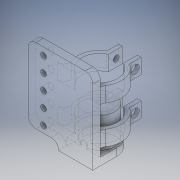
# Autodesk Inventor part: left_motor_mount
Saved by Autodesk Inventor 2018 (Build 220112000, 112)
## iProperties
Created: 2018-03-01
Part Number: left_motor_mount
Material: Generic
Document SubType Name: Modeling
Designer: njcfu
Density: 1 g/cm^3
Appearance: Default
Author: njcfu
Autodesk Inventor part; units mm, degrees
ref_plane "YZ Plane" through (0, 0, 0) normal (1, 0, 0) x (0, 1, 0)
ref_plane "XZ Plane" through (0, 0, 0) normal (0, 1, 0) x (-1, 0, 0)
sketch "Sketch1" plane through (0, 0, 0) normal (0, 1, 0) x (-1, 0, 0)
  circle A0 centre (0, 0) radius 12.7
  dimension "d0" = 25.4
  constraints: 1 centre point, 1 coincident
  measures "d0" diameter of A0
extrude "Extrusion1" add sketch "Sketch1" along normal blind 25.4
ref_plane "Work Plane1" through (0, 0, 12.7) normal (0, 0, 1) x (1, 0, 0)
sketch "Sketch3" plane through (0, 0, 12.7) normal (0, 0, 1) x (1, 0, 0)
  line L0 (-2.5, 0) -> (2.5, 0)
  line L1 (2.5, 0) -> (2.5, 2.4)
  line L2 (2.5, 2.4) -> (-2.5, 2.4)
  line L3 (-2.5, 2.4) -> (-2.5, 0)
  arc A0 (2.5, 2.4) -> (-2.5, 2.4) centre (0, 2.4) ccw
  point P0 (0, 0)
  dimension "d8" = 2.4
  dimension "d9" = 5
  dimension "d10" = 2.5
  dimension "d11" = 2.4
  constraints: 8 end point, 2 parallel, 2 point on circle, 1 centre point, 1 horizontal, 1 midpoint, 1 perpendicular
  measures "d8" distance of L2.end L0.start
  measures "d9" distance of L0.start L0.end
  measures "d10" distance from line of point (0, 0) L3
  measures "d11" distance from line of L2 point (0, 0)
extrude "Extrusion2" add sketch "Sketch3" along normal mid plane 2
sketch "Sketch4" plane through (0, 0, 0) normal (0, -1, 0) x (1, 0, 0)
  line L0 (14.2875, 20.05) -> (-14.2875, 20.05)
  line L1 (-14.2875, 20.05) -> (-14.2875, 0)
  line L2 (14.2875, 0) -> (14.2875, 20.05)
  arc A0 (-14.2875, 0) -> (14.2875, 0) centre (0, 0) ccw
  line L3 (-2.5, 13.7) -> (2.5, 13.7) projected
  arc A1 (-14.2875, 0) -> (14.2875, 0) centre (0, 0) ccw
  line L4 (0, 26.9175) -> (0, -21.155) projected
  circle A2 centre (0, 0) radius 12.7 projected
  dimension "d14" = 6.35
  dimension "d17" = 28.575
  dimension "d18" = 14.2875
  dimension "d19" = 14.2875
  dimension "d20" = 1.5875
  dimension "d21" = 28.575
  constraints: 6 end point, 4 point on circle, 2 centre point, 1 coincident, 1 concentric, 1 horizontal, 1 parallel, 1 perpendicular
  measures "d14" distance between parallel lines of L0 L3
  measures "d17" distance of L0.start L0.end
  measures "d18" distance between parallel lines of L4 L1
  measures "d19" radius of A0
  measures "d20" radial gap between concentric circles of A2 A0
  measures "d21" distance of L2.start L1.end
extrude "Extrusion3" add sketch "Sketch4" along normal blind 6.35
sketch "Sketch5" plane through (0, 0, 0) normal (0, 1, 0) x (1, 0, 0)
  line L0 (-39.6875, -20.05) -> (-39.6875, -13.7)
  line L1 (14.2875, 0) -> (14.2875, -20.05) projected
  line L2 (-39.6875, -20.05) -> (14.2875, -20.05)
  line L3 (14.2875, -20.05) -> (14.2875, -13.7)
  line L4 (14.2875, -13.7) -> (-39.6875, -13.7)
  line L5 (-39.6875, -13.7) -> (-39.6875, -20.05)
  point P0 (0, 0)
  dimension "d22" = 6.35
  dimension "d73" = 53.975
  dimension "d74" = 13.7
  constraints: 10 end point, 2 parallel, 1 horizontal, 1 point on line
  measures "d22" distance between parallel lines of L2 L4
  measures "d73" distance between parallel lines of L0 L1
  measures "d74" distance from line of L1.start L4
extrude "Extrusion4" add sketch "Sketch5" along normal blind 62.7634
ref_plane "Work Plane2" through (0, 12.7, 0) normal (0, -1, 0) x (1, 0, 0)
sketch "Sketch6" plane through (0, 12.7, 0) normal (0, -1, 0) x (1, 0, 0)
  arc A0 (6.35, -13.7142) -> (-6.35, -13.7142) centre (0, 0) ccw
  line L0 (-9.525, -25.4) -> (-9.525, -15.6117)
  line L1 (-4.445, -6.1638) -> (-1.27, -6.1638)
  line L2 (-6.35, -13.7142) -> (-6.35, -25.4)
  line L3 (-6.35, -25.4) -> (-9.525, -25.4)
  line L4 (6.35, -25.4) -> (6.35, -13.7142)
  line L5 (1.6345, -8.3094) -> (4.8095, -8.3094)
  line L6 (9.525, -25.4) -> (6.35, -25.4)
  line L7 (9.525, -15.6117) -> (9.525, -25.4)
  arc A1 (9.525, -15.6117) -> (-9.525, -15.6117) centre (0, 0) ccw
  arc A2 (-14.2875, 0) -> (14.2875, 0) centre (0, 0) ccw projected
  dimension "d26" = 30.226
  dimension "d27" = 3.175
  dimension "d28" = 9.525
  dimension "d29" = 25.4
  dimension "d30" = 3.175
  dimension "d31" = 17.0906
  dimension "d32" = 19.2362
  dimension "d33" = 4.7625
  dimension "d34" = 4.7155
  dimension "d35" = 7.8905
  dimension "d36" = 10.795
  dimension "d37" = 13.97
  constraints: 16 end point, 4 parallel, 4 point on circle, 2 centre point, 2 coincident, 2 equal length, 2 perpendicular, 1 collinear, 1 concentric
  measures "d26" diameter of A0
  measures "d27" distance of L2.end L0.start
  measures "d28" distance from line of point (0, 0) L0
  measures "d29" distance from line of point (0, 0) L3
  measures "d30" radial gap between concentric circles of A0 A1
  measures "d31" distance between parallel lines of L6 L5
  measures "d32" distance between parallel lines of L6 L1
  measures "d33" distance from line of A2.end L7
  measures "d34" distance from line of L5.end L7
  measures "d35" distance from line of L5.start L7
  measures "d36" distance from line of L1.end L7
  measures "d37" distance from line of L1.start L7
extrude "Extrusion5" add sketch "Sketch6" along normal mid plane 12.7
pattern_linear "Rectangular Pattern1" count 2 spacing 31.75 along (0, 1, 0) of "Extrusion5"
sketch "Sketch7" plane through (9.525, 38.1, -15.6117) normal (1, 0, 0) x (0, 0, -1)
  circle A0 centre (4.7083, 6.35) radius 2.4638
  circle A1 centre (4.7083, -25.4) radius 2.4638
  line L0 (9.7883, -31.75) -> (0, -31.75) projected
  line L1 (9.7883, 0) -> (0, 0) projected
  line L2 (9.7883, 12.7) -> (9.7883, 0) projected
  line L3 (9.7883, -19.05) -> (9.7883, -31.75) projected
  point P0 (-15.6117, -38.1)
  dimension "d43" = 4.9276
  dimension "d44" = 4.9276
  dimension "d45" = 6.35
  dimension "d46" = 6.35
  dimension "d47" = 5.08
  dimension "d48" = 5.08
  constraints: 2 centre point
  measures "d43" diameter of A0
  measures "d44" diameter of A1
  measures "d45" distance from line of L0 A1.centre
  measures "d46" distance from line of L1 A0.centre
  measures "d47" distance from line of L2 A0.centre
  measures "d48" distance from line of L3 A1.centre
extrude "Extrusion6" cut sketch "Sketch7" against normal through all
sketch "Sketch8" plane through (9.525, 38.1, -15.6117) normal (1, 0, 0) x (0, 0, -1)
  circle A0 centre (4.7083, 6.35) radius 3.4798
  circle A1 centre (4.7083, -25.4) radius 3.4798
  circle A2 centre (4.7083, 6.35) radius 2.4638 projected
  circle A3 centre (4.7083, -25.4) radius 2.4638 projected
  point P0 (-15.6117, -38.1)
  dimension "d51" = 6.9596
  dimension "d52" = 6.9596
  constraints: 2 centre point, 2 concentric
  measures "d51" diameter of A0
  measures "d52" diameter of A1
extrude "Extrusion7" cut sketch "Sketch8" along normal up to surface (3.175 mm away) from surface at -3.175
fillet "Fillet1" radius 5.08 4 edges at (-12.1145, 44.45, 13.7) (-12.1145, 12.7, 13.7) (12.1145, 44.45, 13.7) (12.1145, 12.7, 13.7)
sketch "Sketch9" plane through (-14.2875, -6.35, 20.05) normal (0, 0, 1) x (1, 0, 0)
  line L0 (0, 6.35) -> (0, 12.7) projected
  circle A0 centre (-12.7, 62.7634) radius 2.4574
  circle A1 centre (-12.7, 50.0634) radius 2.4574
  circle A2 centre (-12.7, 37.3634) radius 2.4574
  circle A3 centre (-12.7, 24.6634) radius 2.4574
  circle A4 centre (-12.7, 11.9634) radius 2.4574
  line L1 (-25.4, 6.35) -> (-25.4, 69.1134) projected
  line L2 (-25.4, 69.1134) -> (28.575, 69.1134) projected
  point P0 (14.2875, 6.35)
  dimension "d56" = 4.9149
  dimension "d57" = 12.7
  dimension "d59" = 12.7
  dimension "d60" = 12.7
  dimension "d61" = 12.7
  dimension "d64" = 4.9149
  dimension "d65" = 4.9149
  dimension "d66" = 4.9149
  dimension "d67" = 4.9149
  dimension "d75" = 12.7
  dimension "d76" = 6.35
  dimension "d77" = 12.7
  dimension "d78" = 12.7
  dimension "d79" = 12.7
  dimension "d80" = 12.7
  constraints: 5 centre point
  measures "d56" diameter of A0
  measures "d57" distance of A0.centre A1.centre
  measures "d59" distance of A2.centre A1.centre
  measures "d60" distance of A3.centre A2.centre
  measures "d61" distance of A3.centre A4.centre
  measures "d64" diameter of A1
  measures "d65" diameter of A2
  measures "d66" diameter of A3
  measures "d67" diameter of A4
  measures "d75" distance from line of L1 A0.centre
  measures "d76" distance from line of L2 A0.centre
  measures "d77" distance from line of L1 A1.centre
  measures "d78" distance from line of L1 A2.centre
  measures "d79" distance from line of L1 A3.centre
  measures "d80" distance from line of L1 A4.centre
extrude "Extrusion8" cut sketch "Sketch9" against normal blind 6.35
fillet "Fillet2" radius 6.35 1 edges at (-14.2875, 0, 16.875)
fillet "Fillet3" radius 6.35 2 edges at (-39.6875, 0, 16.875) (-39.6875, 62.7634, 16.875)
fillet "Fillet4" radius 6.35 1 edges at (14.2875, 62.7634, 16.875)
body "Solid1"
